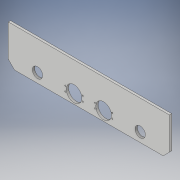
# Autodesk Inventor part: MecanumDriveTrainPlate17-18
Saved by Autodesk Inventor 2017 (Build 210142000, 142)
## iProperties
Created: 2017-09-16
Part Number: MecanumDriveTrainPlate17-18
Material: Generic
Document SubType Name: Modeling
Designer: User
Density: 1 g/cm^3
Appearance: Default
Author: User
Autodesk Inventor part; units mm, degrees
ref_plane "YZ Plane" through (0, 0, 0) normal (1, 0, 0) x (0, 1, 0)
ref_plane "XZ Plane" through (0, 0, 0) normal (0, 1, 0) x (-1, 0, 0)
ref_plane "XY Plane" through (0, 0, 0) normal (0, 0, 1) x (1, 0, 0)
sketch "Sketch1" plane through (0, 0, 0) normal (0, 0, 1) x (1, 0, 0)
  line L0 (0, 0) -> (444.5, 0)
  line L1 (444.5, 0) -> (444.5, 127)
  line L2 (444.5, 127) -> (0, 127)
  line L3 (0, 127) -> (0, 0)
  dimension "d0" = 444.5
  dimension "d1" = 127
  constraints: 8 end point, 2 perpendicular, 1 horizontal, 1 vertical
  measures "d0" distance of L0.start L0.end
  measures "d1" distance of L0.end L1.end
extrude "Extrusion1" add sketch "Sketch1" along normal blind 6.35
sketch "Sketch2" plane through (0, 0, 6.35) normal (0, 0, 1) x (1, 0, 0)
  line L0 (0, 0) -> (444.5, 0) projected
  line L1 (38.0923, 0) -> (0, 38.0919)
  line L2 (0, 127) -> (0, 0) projected
  line L3 (0, 0) -> (444.5, 0) projected
  line L4 (444.5, 0) -> (444.5, 127) projected
  line L5 (444.5, 0) -> (406.4, 0)
  line L6 (444.5, 0) -> (482.6, 0) construction
  line L7 (444.5, 0) -> (444.5, 38.0919)
  line L8 (444.5, 38.0919) -> (406.4086, 0)
  point P0 (419.1126, 0)
  dimension "d19" = 38.1
  dimension "d20" = 180
  constraints: 10 end point, 5 point on line, 3 collinear, 1 horizontal
  measures "d19" distance of L0.end L5.end
  measures "d20" angle of L5 L6
extrude "Extrusion2" cut sketch "Sketch2" against normal blind 50.8
sketch "Sketch3" plane through (0, 0, 6.35) normal (0, 0, 1) x (1, 0, 0)
  line L0 (0, 77.664) -> (80.645, 77.664) construction
  line L1 (444.5, 127) -> (0, 127) projected
  line L2 (80.645, 127) -> (161.29, 127) construction
  circle A0 centre (80.645, 46.355) radius 14.2748
  line L3 (444.5, 38.0919) -> (444.5, 127) projected
  line L4 (444.5, 77.664) -> (525.145, 77.664) construction
  line L5 (444.5, 38.0919) -> (444.5, 127) projected
  line L6 (444.5, 46.355) -> (525.145, 46.355) construction
  circle A1 centre (363.855, 46.355) radius 14.2748
  line L7 (444.5, 127) -> (0, 127) projected
  line L8 (0, 127) -> (0, 38.0919) projected
  circle A2 centre (181.483, 46.355) radius 21.59
  circle A3 centre (263.017, 46.355) radius 21.59
  line L9 (181.483, 46.355) -> (205.486, 46.355)
  line L10 (205.486, 46.355) -> (205.486, 53.3654)
  circle A4 centre (205.486, 53.3654) radius 1.7526
  line L11 (205.486, 46.355) -> (205.486, 39.3446)
  circle A5 centre (205.486, 39.3446) radius 1.7526
  line L12 (181.483, 46.355) -> (157.48, 46.355)
  line L13 (157.48, 46.355) -> (157.48, 53.3654)
  line L14 (157.48, 46.355) -> (157.48, 39.3446)
  circle A6 centre (157.48, 39.3446) radius 1.7526
  circle A7 centre (157.48, 53.3654) radius 1.7526
  line L15 (263.017, 46.355) -> (287.02, 46.355)
  line L16 (263.017, 46.355) -> (239.014, 46.355)
  line L17 (239.014, 46.355) -> (239.014, 53.3654)
  line L18 (239.014, 46.355) -> (239.014, 39.3446)
  line L19 (287.02, 46.355) -> (287.02, 39.3446)
  line L20 (287.02, 46.355) -> (287.02, 53.3654)
  circle A8 centre (287.02, 53.3654) radius 1.7526
  circle A9 centre (287.02, 39.3446) radius 1.7526
  circle A10 centre (239.014, 39.3446) radius 1.7526
  circle A11 centre (239.014, 53.3654) radius 1.7526
  line L21 (263.017, 46.355) -> (256.667, 46.355)
  line L22 (406.4086, 0) -> (444.5, 38.0919) projected
  line L23 (444.5, 38.0919) -> (444.5, 127) projected
  line L24 (444.5, 127) -> (0, 127) projected
  line L25 (0, 127) -> (0, 38.0919) projected
  line L26 (0, 38.0919) -> (38.0923, 0) projected
  line L27 (38.0923, 0) -> (406.4086, 0) projected
  line L28 (406.4086, 0) -> (444.5, 38.0919) projected
  line L29 (444.5, 38.0919) -> (444.5, 127) projected
  line L30 (444.5, 127) -> (0, 127) projected
  line L31 (0, 127) -> (0, 38.0919) projected
  line L32 (0, 38.0919) -> (38.0923, 0) projected
  line L33 (38.0923, 0) -> (406.4086, 0) projected
  line L34 (38.0923, 0) -> (0, 38.0919) projected
  line L35 (0, 38.0919) -> (0, 127) projected
  line L36 (0, 127) -> (444.5, 127) projected
  line L37 (444.5, 127) -> (444.5, 38.0919) projected
  line L38 (444.5, 38.0919) -> (406.4086, 0) projected
  line L39 (406.4086, 0) -> (38.0923, 0) projected
  point P0 (0, 0)
  dimension "d10" = 28.5496
  dimension "d18" = 28.5496
  dimension "d31" = 43.18
  dimension "d32" = 43.18
  dimension "d55" = 24.003
  dimension "d56" = 7.0104
  dimension "d57" = 3.5052
  dimension "d58" = 7.0104
  dimension "d59" = 3.5052
  dimension "d60" = 24.003
  dimension "d61" = 7.0104
  dimension "d62" = 7.0104
  dimension "d63" = 3.5052
  dimension "d64" = 3.5052
  dimension "d65" = 24.003
  dimension "d66" = 24.003
  dimension "d67" = 3.5052
  dimension "d68" = 3.5052
  dimension "d69" = 3.5052
  dimension "d70" = 3.5052
  dimension "d73" = 6.35
  dimension "d74" = 181.483
  dimension "d75" = 181.483
  constraints: 34 end point, 12 centre point, 9 coincident, 8 horizontal, 6 vertical, 4 point on line, 2 perpendicular
  measures "d10" diameter of A0
  measures "d18" diameter of A1
  measures "d31" diameter of A2
  measures "d32" diameter of A3
  measures "d55" distance of L9.start L9.end
  measures "d56" distance of L9.end L10.end
  measures "d57" diameter of A4
  measures "d58" distance of L9.end L11.end
  measures "d59" diameter of A5
  measures "d60" distance of L9.start L12.end
  measures "d61" distance of L12.end L13.end
  measures "d62" distance of L12.end L14.end
  measures "d63" diameter of A6
  measures "d64" diameter of A7
  measures "d65" distance of L15.start L15.end
  measures "d66" distance of L15.start L16.end
  measures "d67" diameter of A8
  measures "d68" diameter of A9
  measures "d69" diameter of A10
  measures "d70" diameter of A11
  measures "d73" distance of L15.start L21.end
  measures "d74" distance from line of L8 L9.start
  measures "d75" distance from line of L5 L15.start
extrude "Extrusion3" cut sketch "Sketch3" against normal blind 50.8 contours A0 | A1
extrude "Extrusion4" cut sketch "Sketch3" against normal blind 25.4 contours L9 L12 A2 | A2 L12 L9 | L15 L16 A3 | A3 L16 L15
thicken "Thicken1" operation add thickness 20.828 both sides no extend neighbours yes toward (0, 1, 0) faces at (160.8644, 0, 2.1167)
extrude "Extrusion6" cut sketch "Sketch3" against normal blind 25.4 contours A4 | A5 | A6 | A7 | A8 | A9 | A10 | A11
body "Solid1"
